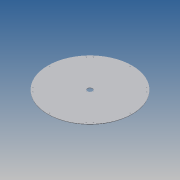
# Autodesk Inventor part: 2f1bd
Saved by Autodesk Inventor 2014 SP1 (Build 180222100, 222)
## iProperties
Company: HERA Project
Created: 2013-05-22
Part Number: 2f1bd
Material: Aluminum 6061
Document SubType Name: Modeling
Designer: Rich Bradley
Density: 2.71 g/cm^3
Description: Feed bottom disk
Mass: 2472.03 g
Surface Area: 5814.47 cm^2
Volume: 912.187 cm^3
Appearance: Aluminum - Flat
Translation Standard: STEP AP214IS
FileName: C:/Users/Dave/Desktop/PAPER/paperElement.step
PostProcessor: Build: 138, Release: 2013 RTM - Date: Thu 03/01/2012
Sent Units: millimeter
Uncertainty: 2.54e-05
Author: David DeBoer
Title: Feed bottom disk
Autodesk Inventor part; units mm, degrees
ref_plane "YZ Plane" through (0, 0, 0) normal (1, 0, 0) x (0, 1, 0)
ref_plane "XZ Plane" through (0, 0, 0) normal (0, 1, 0) x (-1, 0, 0)
ref_plane "XY Plane" through (0, 0, 0) normal (0, 0, 1) x (1, 0, 0)
sketch "Sketch1" plane through (0, 0, 0) normal (0, 1, 0) x (-1, 0, 0)
  circle A0 centre (0, 0) radius 304.8
  dimension "d0" = 609.6
  constraints: 1 centre point, 1 coincident
  measures "d0" diameter of A0
extrude "Extrusion1" add sketch "Sketch1" along normal blind 3.175
sketch "Sketch2" plane through (0, 3.175, 0) normal (0, 1, 0) x (1, 0, 0)
  circle A0 centre (0, 0) radius 304.8 projected
  circle A1 centre (0, 0) radius 19.05
  dimension "d3" = 38.1
  constraints: 1 centre point, 1 coincident
  measures "d3" diameter of A1
extrude "Extrusion2" cut sketch "Sketch2" against normal blind 3.175 contours A1
sketch "Sketch3" plane through (0, 3.175, 0) normal (0, 1, 0) x (1, 0, 0)
  circle A0 centre (0, 0) radius 19.05 projected
  circle A1 centre (0, 292.1) radius 4.6302
  dimension "d6" = 292.1
  constraints: 1 centre point
  measures "d6" distance of A1.centre A0.centre
hole "Hole1" at (0, 3.175, -292.1) direction (0, -1, 0) diameter 4.4958 end through all countersink diameter 8.4328 countersink angle 82
pattern_circular "Circular Pattern1" count 4 over 360 about axis through (0, 3.175, 0) along (0, -1, 0) of "Hole1"
sketch "Sketch4" plane through (0, 3.175, 0) normal (0, 1, 0) x (1, 0, 0)
  circle A0 centre (0, 0) radius 304.8 projected
  line L0 (0, 0) -> (304.8, 0) construction
  line L1 (0, 0) -> (206.5459, 206.5459) construction
  line L2 (193.6323, 219.4595) -> (-44.0898, -18.2626) construction
  line L3 (-44.0898, -18.2626) -> (304.8, -18.2626) construction
  line L4 (219.4595, 193.6323) -> (44.0898, 18.2626) construction
  line L5 (44.0898, 18.2626) -> (304.8, 18.2626) construction
  circle A1 centre (193.6323, 219.4595) radius 4.0648
  circle A2 centre (219.4595, 193.6323) radius 4.0772
  dimension "d20" = 292.1
  dimension "d21" = 45
  dimension "d22" = 18.2626
  dimension "d23" = 18.2626
  constraints: 12 end point, 2 centre point, 2 coincident, 1 horizontal, 1 horizontal alignment, 3 other
  measures "d20" distance of L0.start L1.end
  measures "d21" angle of L0 L1
  measures "d22" distance between parallel lines of L1 L2
  measures "d23" distance between parallel lines of L4 L1
hole "Hole2" at (193.6323, 3.175, -219.4595) at (219.4595, 3.175, -193.6323) direction (0, -1, 0) diameter 4.4958 end through all countersink diameter 8.4328 countersink angle 82
pattern_circular "Circular Pattern2" count 4 over 360 about axis through (0, 3.175, 0) along (0, -1, 0) of "Hole2"
sketch "Sketch5" plane through (0, 3.175, 0) normal (0, 1, 0) x (1, 0, 0)
  circle A0 centre (0, 0) radius 19.05 projected
  circle A1 centre (0, 22.225) radius 4.7781
  dimension "d34" = 22.225
  constraints: 1 centre point
  measures "d34" distance of A0.centre A1.centre
hole "Hole3" at (0, 3.175, -22.225) direction (0, -1, 0) diameter 2.438 depth 8 tip angle 118 clearance for "Flat Head Machine Screw (82)" size "#2" standard "Ansi Unified Screw Threads"
pattern_circular "Circular Pattern3" count 4 over 360 about axis through (0, 3.175, 0) along (0, -1, 0) of "Hole3"
body "Solid2"
